Autodesk Fusion 360 part; units mm, degrees
(part 2 of 2)
  arc A18 (-11.9213, -3.7594) -> (-11.7413, -4.2886) centre (0, 0) ccw
  spline S37 degree 5 poles (-11.7413, -4.2886) (-11.7404, -4.3045) (-11.7391, -4.3362) (-11.7389, -4.383) (-11.7421, -4.4438) (-11.7524, -4.517) (-11.7695, -4.5872) (-11.7939, -4.6541) (-11.8261, -4.7177) (-11.8656, -4.778) (-11.9119, -4.8353) (-11.954, -4.8789) (-11.9882, -4.9104) (-12.0121, -4.931) (-12.0244, -4.9411) knots -1 -1 -1 -1 -1 -1 -0.9 -0.8 -0.7 -0.6 -0.5 -0.4 -0.3 -0.2 -0.1 0 0 0 0 0 0
  line L95 (-12.0244, -4.9411) -> (-12.9493, -5.3212)
  line L96 (-12.9493, -5.3212) -> (-14.2037, -6.215)
  line L97 (-14.2037, -6.215) -> (-13.8236, -7.14)
  line L98 (-13.8236, -7.14) -> (-12.2495, -6.8715)
  line L99 (-12.2495, -6.8715) -> (-11.2708, -6.4694)
  spline S38 degree 5 poles (-11.2708, -6.4694) (-11.2543, -6.467) (-11.2214, -6.4628) (-11.1727, -6.4584) (-11.1087, -6.4566) (-11.0305, -6.4612) (-10.9543, -6.4735) (-10.8803, -6.494) (-10.8086, -6.523) (-10.739, -6.5603) (-10.6714, -6.6051) (-10.6188, -6.6465) (-10.5801, -6.6805) (-10.5547, -6.7045) (-10.542, -6.7168) knots 0 0 0 0 0 0 0.1 0.2 0.3 0.4 0.5 0.6 0.7 0.8 0.9 1 1 1 1 1 1
  arc A19 (-10.542, -6.7168) -> (-10.2313, -7.1813) centre (0, 0) ccw
  spline S39 degree 5 poles (-10.2313, -7.1813) (-10.2262, -7.1965) (-10.2168, -7.2268) (-10.2045, -7.2719) (-10.1918, -7.3314) (-10.1828, -7.4048) (-10.1812, -7.477) (-10.1875, -7.548) (-10.2021, -7.6177) (-10.2246, -7.6862) (-10.2546, -7.7535) (-10.2839, -7.8066) (-10.3088, -7.8459) (-10.3266, -7.8719) (-10.3358, -7.8849) knots -1 -1 -1 -1 -1 -1 -0.9 -0.8 -0.7 -0.6 -0.5 -0.4 -0.3 -0.2 -0.1 0 0 0 0 0 0
  line L100 (-10.3358, -7.8849) -> (-11.1309, -8.4914)
  line L101 (-11.1309, -8.4914) -> (-12.1112, -9.6795)
  line L102 (-12.1112, -9.6795) -> (-11.5047, -10.4745)
  line L103 (-11.5047, -10.4745) -> (-10.0536, -9.8078)
  line L104 (-10.0536, -9.8078) -> (-9.2124, -9.166)
  spline S40 degree 5 poles (-9.2124, -9.166) (-9.197, -9.1594) (-9.1664, -9.1469) (-9.1204, -9.1301) (-9.0591, -9.1117) (-8.9823, -9.096) (-8.9056, -9.0881) (-8.8288, -9.0888) (-8.752, -9.0982) (-8.6752, -9.1162) (-8.5983, -9.142) (-8.5367, -9.1684) (-8.4906, -9.1913) (-8.4598, -9.2078) (-8.4444, -9.2164) knots 0 0 0 0 0 0 0.1 0.2 0.3 0.4 0.5 0.6 0.7 0.8 0.9 1 1 1 1 1 1
  arc A20 (-8.4444, -9.2164) -> (-8.024, -9.5847) centre (0, 0) ccw
  spline S41 degree 5 poles (-8.024, -9.5847) (-8.0152, -9.598) (-7.9982, -9.6248) (-7.9747, -9.6652) (-7.9471, -9.7194) (-7.9194, -9.788) (-7.8991, -9.8573) (-7.8868, -9.9276) (-7.8828, -9.9987) (-7.8869, -10.0706) (-7.8984, -10.1434) (-7.913, -10.2022) (-7.9268, -10.2466) (-7.9373, -10.2764) (-7.9429, -10.2913) knots -1 -1 -1 -1 -1 -1 -0.9 -0.8 -0.7 -0.6 -0.5 -0.4 -0.3 -0.2 -0.1 0 0 0 0 0 0
  line L105 (-7.9429, -10.2913) -> (-8.5539, -11.0829)
  line L106 (-8.5539, -11.0829) -> (-9.1933, -12.4842)
  line L107 (-9.1933, -12.4842) -> (-8.4016, -13.0952)
  line L108 (-8.4016, -13.0952) -> (-7.1726, -12.0756)
  line L109 (-7.1726, -12.0756) -> (-6.5261, -11.238)
  spline S42 degree 5 poles (-6.5261, -11.238) (-6.513, -11.2277) (-6.4867, -11.2076) (-6.4466, -11.1795) (-6.3921, -11.1459) (-6.3221, -11.1109) (-6.25, -11.0834) (-6.1756, -11.0641) (-6.099, -11.0534) (-6.0201, -11.0509) (-5.9392, -11.0559) (-5.8729, -11.0655) (-5.8224, -11.0756) (-5.7884, -11.0836) (-5.7713, -11.0879) knots 0 0 0 0 0 0 0.1 0.2 0.3 0.4 0.5 0.6 0.7 0.8 0.9 1 1 1 1 1 1
  arc A21 (-5.7713, -11.0879) -> (-5.2699, -11.3348) centre (0, 0) ccw
  spline S43 degree 5 poles (-5.2699, -11.3348) (-5.2579, -11.3455) (-5.2346, -11.3669) (-5.2014, -11.3998) (-5.1607, -11.4451) (-5.1162, -11.5042) (-5.0786, -11.5659) (-5.0486, -11.6305) (-5.0264, -11.6982) (-5.0117, -11.7688) (-5.0039, -11.842) (-5.0029, -11.9026) (-5.0047, -11.9491) (-5.0071, -11.9806) (-5.0086, -11.9964) knots -1 -1 -1 -1 -1 -1 -0.9 -0.8 -0.7 -0.6 -0.5 -0.4 -0.3 -0.2 -0.1 0 0 0 0 0 0
  line L110 (-5.0086, -11.9964) -> (-5.3939, -12.9192)
  line L111 (-5.3939, -12.9192) -> (-5.6489, -14.4382)
  line L112 (-5.6489, -14.4382) -> (-4.7261, -14.8235)
  line L113 (-4.7261, -14.8235) -> (-3.8028, -13.5206)
  line L114 (-3.8028, -13.5206) -> (-3.3951, -12.5442)
  spline S44 degree 5 poles (-3.3951, -12.5442) (-3.3852, -12.5308) (-3.3649, -12.5046) (-3.3335, -12.4671) (-3.2895, -12.4205) (-3.2309, -12.3685) (-3.1684, -12.3233) (-3.1016, -12.2855) (-3.0303, -12.2553) (-2.9548, -12.2325) (-2.8753, -12.2164) (-2.8088, -12.2085) (-2.7574, -12.2051) (-2.7225, -12.2041) (-2.7049, -12.2038) knots 0 0 0 0 0 0 0.1 0.2 0.3 0.4 0.5 0.6 0.7 0.8 0.9 1 1 1 1 1 1
  arc A22 (-2.7049, -12.2038) -> (-2.1566, -12.3126) centre (0, 0) ccw
  spline S45 degree 5 poles (-2.1566, -12.3126) (-2.1423, -12.3197) (-2.1143, -12.3344) (-2.0737, -12.3576) (-2.0226, -12.3908) (-1.9644, -12.4363) (-1.9121, -12.4862) (-1.8664, -12.5409) (-1.8274, -12.6005) (-1.7949, -12.6649) (-1.7685, -12.7337) (-1.7518, -12.7919) (-1.7415, -12.8373) (-1.7357, -12.8683) (-1.7331, -12.884) knots -1 -1 -1 -1 -1 -1 -0.9 -0.8 -0.7 -0.6 -0.5 -0.4 -0.3 -0.2 -0.1 0 0 0 0 0 0
  line L115 (-1.7331, -12.884) -> (-1.8664, -13.875)
  line L116 (-1.8664, -13.875) -> (-1.7195, -15.4083)
  line L117 (-1.7195, -15.4083) -> (-0.7284, -15.5416)
  line L118 (-0.7284, -15.5416) -> (-0.1738, -14.0441)
  line L119 (-0.1738, -14.0441) -> (0, -12.7519)
  line L120 (0, -12.7519) -> (0, -12.9212)
  spline S46 degree 5 poles (0, -12.9212) (0.0001, -12.921) (0.0073, -12.9063) (0.0221, -12.8775) (0.0458, -12.8358) (0.0804, -12.7833) (0.1291, -12.7235) (0.1838, -12.6697) (0.2448, -12.622) (0.3119, -12.5804) (0.3845, -12.5443) (0.4467, -12.5194) (0.4955, -12.5029) (0.5289, -12.4929) (0.5459, -12.4881) knots 0.098741 0.098741 0.098741 0.098741 0.098741 0.098741 0.1 0.2 0.3 0.4 0.5 0.6 0.7 0.8 0.9 1 1 1 1 1 1
  arc A23 (0.5459, -12.4881) -> (1.1036, -12.4512) centre (0, 0) ccw
  spline S47 degree 5 poles (1.1036, -12.4512) (1.1192, -12.4544) (1.1502, -12.4614) (1.1954, -12.4733) (1.2533, -12.4921) (1.3213, -12.521) (1.3847, -12.5557) (1.443, -12.5966) (1.4961, -12.6441) (1.5441, -12.6979) (1.5875, -12.7575) (1.6187, -12.8094) (1.6403, -12.8506) (1.654, -12.879) (1.6606, -12.8935) knots -1 -1 -1 -1 -1 -1 -0.9 -0.8 -0.7 -0.6 -0.5 -0.4 -0.3 -0.2 -0.1 0 0 0 0 0 0
  line L121 (1.6606, -12.8935) -> (1.7883, -13.8853)
  line L122 (1.7883, -13.8853) -> (2.3271, -15.3283)
  circle A24 centre (0, 0) radius 1.5
  dimension "d23" = 3
  constraint coincident A0.centre A1.centre
  measures "d23" diameter of A24
extrude "Extrude2" cut sketch "Sketch2" against normal blind 10 contours A24
sketch "Sketch3" plane through (0, 4, 0) normal (0, 1, 0) x (-1, 0, 0)
  circle A0 centre (0, 0) radius 1.5
  line L0 (2.3271, -15.3283) -> (3.3189, -15.2006)
  line L1 (3.3189, -15.2006) -> (3.467, -13.6106)
  line L2 (3.467, -13.6106) -> (3.3318, -12.5612)
  spline S0 degree 5 poles (3.3318, -12.5612) (3.3338, -12.5446) (3.3382, -12.5118) (3.3467, -12.4635) (3.3614, -12.4012) (3.3862, -12.3269) (3.4177, -12.2565) (3.4567, -12.1904) (3.5033, -12.1286) (3.5573, -12.071) (3.6181, -12.0173) (3.6717, -11.9772) (3.7146, -11.9487) (3.7443, -11.9303) (3.7594, -11.9213) knots 0 0 0 0 0 0 0.1 0.2 0.3 0.4 0.5 0.6 0.7 0.8 0.9 1 1 1 1 1 1
  arc A1 (3.7594, -11.9213) -> (4.751, -11.5619) centre (0, 0) ccw
  line L3 (4.751, -11.5619) -> (4.3177, -11.74)
  spline S1 degree 5 poles (4.3177, -11.74) (4.3277, -11.7396) (4.3533, -11.7391) (4.3941, -11.7395) (4.4491, -11.7428) (4.517, -11.7524) (4.5872, -11.7695) (4.6541, -11.7939) (4.7177, -11.8261) (4.778, -11.8656) (4.8353, -11.9119) (4.8789, -11.954) (4.9104, -11.9882) (4.931, -12.0121) (4.9411, -12.0244) knots -0.963292 -0.963292 -0.963292 -0.963292 -0.963292 -0.963292 -0.9 -0.8 -0.7 -0.6 -0.5 -0.4 -0.3 -0.2 -0.1 0 0 0 0 0 0
  line L4 (4.9411, -12.0244) -> (5.3212, -12.9493)
  line L5 (5.3212, -12.9493) -> (6.215, -14.2037)
  line L6 (6.215, -14.2037) -> (7.14, -13.8236)
  line L7 (7.14, -13.8236) -> (6.8715, -12.2495)
  line L8 (6.8715, -12.2495) -> (6.4694, -11.2708)
  spline S2 degree 5 poles (6.4694, -11.2708) (6.467, -11.2543) (6.4628, -11.2214) (6.4584, -11.1727) (6.4566, -11.1087) (6.4612, -11.0305) (6.4735, -10.9543) (6.494, -10.8803) (6.523, -10.8086) (6.5603, -10.739) (6.6013, -10.6771) (6.6378, -10.63) (6.6663, -10.5966) (6.6845, -10.5763) (6.6913, -10.569) knots 0 0 0 0 0 0 0.1 0.2 0.3 0.4 0.5 0.6 0.7 0.8 0.9 0.957627 0.957627 0.957627 0.957627 0.957627 0.957627
  line L9 (6.6913, -10.569) -> (6.2793, -10.8083)
  arc A2 (6.2793, -10.8083) -> (7.1813, -10.2313) centre (0, 0) ccw
  spline S3 degree 5 poles (7.1813, -10.2313) (7.1965, -10.2262) (7.2268, -10.2168) (7.2719, -10.2045) (7.3314, -10.1918) (7.4048, -10.1828) (7.477, -10.1812) (7.548, -10.1875) (7.6177, -10.2021) (7.6862, -10.2246) (7.7535, -10.2546) (7.8066, -10.2839) (7.8459, -10.3088) (7.8719, -10.3266) (7.8849, -10.3358) knots -1 -1 -1 -1 -1 -1 -0.9 -0.8 -0.7 -0.6 -0.5 -0.4 -0.3 -0.2 -0.1 0 0 0 0 0 0
  line L10 (7.8849, -10.3358) -> (8.4914, -11.1309)
  line L11 (8.4914, -11.1309) -> (9.6795, -12.1112)
  line L12 (9.6795, -12.1112) -> (10.4745, -11.5047)
  line L13 (10.4745, -11.5047) -> (9.8078, -10.0536)
  line L14 (9.8078, -10.0536) -> (9.166, -9.2124)
  spline S4 degree 5 poles (9.166, -9.2124) (9.1594, -9.197) (9.1469, -9.1664) (9.1301, -9.1204) (9.1117, -9.0591) (9.096, -8.9823) (9.0881, -8.9056) (9.0888, -8.8288) (9.0982, -8.752) (9.1162, -8.6752) (9.142, -8.5983) (9.1684, -8.5367) (9.1913, -8.4906) (9.2078, -8.4598) (9.2164, -8.4444) knots 0 0 0 0 0 0 0.1 0.2 0.3 0.4 0.5 0.6 0.7 0.8 0.9 1 1 1 1 1 1
  arc A3 (9.2164, -8.4444) -> (9.5847, -8.024) centre (0, 0) ccw
  spline S5 degree 5 poles (9.5847, -8.024) (9.598, -8.0152) (9.6248, -7.9982) (9.6652, -7.9747) (9.7194, -7.9471) (9.788, -7.9194) (9.8573, -7.8991) (9.9276, -7.8868) (9.9987, -7.8828) (10.0706, -7.8869) (10.1434, -7.8984) (10.2022, -7.913) (10.2466, -7.9268) (10.2764, -7.9373) (10.2913, -7.9429) knots -1 -1 -1 -1 -1 -1 -0.9 -0.8 -0.7 -0.6 -0.5 -0.4 -0.3 -0.2 -0.1 0 0 0 0 0 0
  line L15 (10.2913, -7.9429) -> (11.0829, -8.5539)
  line L16 (11.0829, -8.5539) -> (12.4842, -9.1933)
  line L17 (12.4842, -9.1933) -> (13.0952, -8.4016)
  line L18 (13.0952, -8.4016) -> (12.0756, -7.1726)
  line L19 (12.0756, -7.1726) -> (11.238, -6.5261)
  spline S6 degree 5 poles (11.238, -6.5261) (11.2277, -6.513) (11.2076, -6.4867) (11.1795, -6.4466) (11.1459, -6.3921) (11.1109, -6.3221) (11.0834, -6.25) (11.0641, -6.1756) (11.0534, -6.099) (11.0509, -6.0201) (11.0559, -5.9392) (11.0655, -5.8729) (11.0756, -5.8224) (11.0836, -5.7884) (11.0879, -5.7713) knots 0 0 0 0 0 0 0.1 0.2 0.3 0.4 0.5 0.6 0.7 0.8 0.9 1 1 1 1 1 1
  arc A4 (11.0879, -5.7713) -> (11.3348, -5.2699) centre (0, 0) ccw
  spline S7 degree 5 poles (11.3348, -5.2699) (11.3455, -5.2579) (11.3669, -5.2346) (11.3998, -5.2014) (11.4451, -5.1607) (11.5042, -5.1162) (11.5659, -5.0786) (11.6305, -5.0486) (11.6982, -5.0264) (11.7688, -5.0117) (11.842, -5.0039) (11.9026, -5.0029) (11.9491, -5.0047) (11.9806, -5.0071) (11.9964, -5.0086) knots -1 -1 -1 -1 -1 -1 -0.9 -0.8 -0.7 -0.6 -0.5 -0.4 -0.3 -0.2 -0.1 0 0 0 0 0 0
  line L20 (11.9964, -5.0086) -> (12.9192, -5.3939)
  line L21 (12.9192, -5.3939) -> (14.4382, -5.6489)
  line L22 (14.4382, -5.6489) -> (14.8235, -4.7261)
  line L23 (14.8235, -4.7261) -> (13.5206, -3.8028)
  line L24 (13.5206, -3.8028) -> (12.5442, -3.3951)
  spline S8 degree 5 poles (12.5442, -3.3951) (12.5308, -3.3852) (12.5046, -3.3649) (12.4671, -3.3335) (12.4205, -3.2895) (12.3685, -3.2309) (12.3233, -3.1684) (12.2855, -3.1016) (12.2553, -3.0303) (12.2325, -2.9548) (12.2164, -2.8753) (12.2085, -2.8088) (12.2051, -2.7574) (12.2041, -2.7225) (12.2038, -2.7049) knots 0 0 0 0 0 0 0.1 0.2 0.3 0.4 0.5 0.6 0.7 0.8 0.9 1 1 1 1 1 1
  arc A5 (12.2038, -2.7049) -> (12.3126, -2.1566) centre (0, 0) ccw
  spline S9 degree 5 poles (12.3126, -2.1566) (12.3197, -2.1423) (12.3344, -2.1143) (12.3576, -2.0737) (12.3908, -2.0226) (12.4363, -1.9644) (12.4862, -1.9121) (12.5409, -1.8664) (12.6005, -1.8274) (12.6649, -1.7949) (12.7337, -1.7685) (12.7919, -1.7518) (12.8373, -1.7415) (12.8683, -1.7357) (12.884, -1.7331) knots -1 -1 -1 -1 -1 -1 -0.9 -0.8 -0.7 -0.6 -0.5 -0.4 -0.3 -0.2 -0.1 0 0 0 0 0 0
  line L25 (12.884, -1.7331) -> (13.875, -1.8664)
  line L26 (13.875, -1.8664) -> (15.4083, -1.7195)
  line L27 (15.4083, -1.7195) -> (15.5416, -0.7284)
  line L28 (15.5416, -0.7284) -> (14.0441, -0.1738)
  line L29 (14.0441, -0.1738) -> (12.9955, -0.0328)
  spline S10 degree 5 poles (12.9955, -0.0328) (12.98, -0.0266) (12.9494, -0.0138) (12.905, 0.0068) (12.8487, 0.0372) (12.7833, 0.0804) (12.7235, 0.1291) (12.6697, 0.1838) (12.622, 0.2448) (12.5804, 0.3119) (12.5443, 0.3845) (12.5194, 0.4467) (12.5029, 0.4955) (12.4929, 0.5289) (12.4881, 0.5459) knots 0 0 0 0 0 0 0.1 0.2 0.3 0.4 0.5 0.6 0.7 0.8 0.9 1 1 1 1 1 1
  arc A6 (12.4881, 0.5459) -> (12.4512, 1.1036) centre (0, 0) ccw
  spline S11 degree 5 poles (12.4512, 1.1036) (12.4544, 1.1192) (12.4614, 1.1502) (12.4733, 1.1954) (12.4921, 1.2533) (12.521, 1.3213) (12.5557, 1.3847) (12.5966, 1.443) (12.6441, 1.4961) (12.6979, 1.5441) (12.7575, 1.5875) (12.8094, 1.6187) (12.8506, 1.6403) (12.879, 1.654) (12.8935, 1.6606) knots -1 -1 -1 -1 -1 -1 -0.9 -0.8 -0.7 -0.6 -0.5 -0.4 -0.3 -0.2 -0.1 0 0 0 0 0 0
  line L30 (12.8935, 1.6606) -> (13.8853, 1.7883)
  line L31 (13.8853, 1.7883) -> (15.3283, 2.3271)
  line L32 (15.3283, 2.3271) -> (15.2006, 3.3189)
  line L33 (15.2006, 3.3189) -> (13.6106, 3.467)
  line L34 (13.6106, 3.467) -> (12.5612, 3.3318)
  spline S12 degree 5 poles (12.5612, 3.3318) (12.5446, 3.3338) (12.5118, 3.3382) (12.4635, 3.3467) (12.4012, 3.3614) (12.3269, 3.3862) (12.2565, 3.4177) (12.1904, 3.4567) (12.1286, 3.5033) (12.071, 3.5573) (12.0173, 3.6181) (11.9772, 3.6717) (11.9487, 3.7146) (11.9303, 3.7443) (11.9213, 3.7594) knots 0 0 0 0 0 0 0.1 0.2 0.3 0.4 0.5 0.6 0.7 0.8 0.9 1 1 1 1 1 1
  arc A7 (11.9213, 3.7594) -> (11.7413, 4.2886) centre (0, 0) ccw
  spline S13 degree 5 poles (11.7413, 4.2886) (11.7404, 4.3045) (11.7391, 4.3362) (11.7389, 4.383) (11.7421, 4.4438) (11.7524, 4.517) (11.7695, 4.5872) (11.7939, 4.6541) (11.8261, 4.7177) (11.8656, 4.778) (11.9119, 4.8353) (11.954, 4.8789) (11.9882, 4.9104) (12.0121, 4.931) (12.0244, 4.9411) knots -1 -1 -1 -1 -1 -1 -0.9 -0.8 -0.7 -0.6 -0.5 -0.4 -0.3 -0.2 -0.1 0 0 0 0 0 0
  line L35 (12.0244, 4.9411) -> (12.9493, 5.3212)
  line L36 (12.9493, 5.3212) -> (14.2037, 6.215)
  line L37 (14.2037, 6.215) -> (13.8236, 7.14)
  line L38 (13.8236, 7.14) -> (12.2495, 6.8715)
  line L39 (12.2495, 6.8715) -> (11.2708, 6.4694)
  spline S14 degree 5 poles (11.2708, 6.4694) (11.2543, 6.467) (11.2214, 6.4628) (11.1727, 6.4584) (11.1087, 6.4566) (11.0305, 6.4612) (10.9543, 6.4735) (10.8803, 6.494) (10.8086, 6.523) (10.739, 6.5603) (10.6714, 6.6051) (10.6188, 6.6465) (10.5801, 6.6805) (10.5547, 6.7045) (10.542, 6.7168) knots 0 0 0 0 0 0 0.1 0.2 0.3 0.4 0.5 0.6 0.7 0.8 0.9 1 1 1 1 1 1
  arc A8 (10.542, 6.7168) -> (10.2313, 7.1813) centre (0, 0) ccw
  spline S15 degree 5 poles (10.2313, 7.1813) (10.2262, 7.1965) (10.2168, 7.2268) (10.2045, 7.2719) (10.1918, 7.3314) (10.1828, 7.4048) (10.1812, 7.477) (10.1875, 7.548) (10.2021, 7.6177) (10.2246, 7.6862) (10.2546, 7.7535) (10.2839, 7.8066) (10.3088, 7.8459) (10.3266, 7.8719) (10.3358, 7.8849) knots -1 -1 -1 -1 -1 -1 -0.9 -0.8 -0.7 -0.6 -0.5 -0.4 -0.3 -0.2 -0.1 0 0 0 0 0 0
  line L40 (10.3358, 7.8849) -> (11.1309, 8.4914)
  line L41 (11.1309, 8.4914) -> (12.1112, 9.6795)
  line L42 (12.1112, 9.6795) -> (11.5047, 10.4745)
  line L43 (11.5047, 10.4745) -> (10.0536, 9.8078)
  line L44 (10.0536, 9.8078) -> (9.2124, 9.166)
  spline S16 degree 5 poles (9.2124, 9.166) (9.197, 9.1594) (9.1664, 9.1469) (9.1204, 9.1301) (9.0591, 9.1117) (8.9823, 9.096) (8.9056, 9.0881) (8.8288, 9.0888) (8.752, 9.0982) (8.6752, 9.1162) (8.5983, 9.142) (8.5367, 9.1684) (8.4906, 9.1913) (8.4598, 9.2078) (8.4444, 9.2164) knots 0 0 0 0 0 0 0.1 0.2 0.3 0.4 0.5 0.6 0.7 0.8 0.9 1 1 1 1 1 1
  arc A9 (8.4444, 9.2164) -> (8.024, 9.5847) centre (0, 0) ccw
  spline S17 degree 5 poles (8.024, 9.5847) (8.0152, 9.598) (7.9982, 9.6248) (7.9747, 9.6652) (7.9471, 9.7194) (7.9194, 9.788) (7.8991, 9.8573) (7.8868, 9.9276) (7.8828, 9.9987) (7.8869, 10.0706) (7.8984, 10.1434) (7.913, 10.2022) (7.9268, 10.2466) (7.9373, 10.2764) (7.9429, 10.2913) knots -1 -1 -1 -1 -1 -1 -0.9 -0.8 -0.7 -0.6 -0.5 -0.4 -0.3 -0.2 -0.1 0 0 0 0 0 0
  line L45 (7.9429, 10.2913) -> (8.5539, 11.0829)
  line L46 (8.5539, 11.0829) -> (9.1933, 12.4842)
  line L47 (9.1933, 12.4842) -> (8.4016, 13.0952)
  line L48 (8.4016, 13.0952) -> (7.1726, 12.0756)
  line L49 (7.1726, 12.0756) -> (6.5261, 11.238)
  spline S18 degree 5 poles (6.5261, 11.238) (6.513, 11.2277) (6.4867, 11.2076) (6.4466, 11.1795) (6.3921, 11.1459) (6.3221, 11.1109) (6.25, 11.0834) (6.1756, 11.0641) (6.099, 11.0534) (6.0201, 11.0509) (5.9392, 11.0559) (5.8729, 11.0655) (5.8224, 11.0756) (5.7884, 11.0836) (5.7713, 11.0879) knots 0 0 0 0 0 0 0.1 0.2 0.3 0.4 0.5 0.6 0.7 0.8 0.9 1 1 1 1 1 1
  arc A10 (5.7713, 11.0879) -> (5.2699, 11.3348) centre (0, 0) ccw
  spline S19 degree 5 poles (5.2699, 11.3348) (5.2579, 11.3455) (5.2346, 11.3669) (5.2014, 11.3998) (5.1607, 11.4451) (5.1162, 11.5042) (5.0786, 11.5659) (5.0486, 11.6305) (5.0264, 11.6982) (5.0117, 11.7688) (5.0039, 11.842) (5.0029, 11.9026) (5.0047, 11.9491) (5.0071, 11.9806) (5.0086, 11.9964) knots -1 -1 -1 -1 -1 -1 -0.9 -0.8 -0.7 -0.6 -0.5 -0.4 -0.3 -0.2 -0.1 0 0 0 0 0 0
  line L50 (5.0086, 11.9964) -> (5.3939, 12.9192)
  line L51 (5.3939, 12.9192) -> (5.6489, 14.4382)
  line L52 (5.6489, 14.4382) -> (4.7261, 14.8235)
  line L53 (4.7261, 14.8235) -> (3.8028, 13.5206)
  line L54 (3.8028, 13.5206) -> (3.3951, 12.5442)
  spline S20 degree 5 poles (3.3951, 12.5442) (3.3852, 12.5308) (3.3649, 12.5046) (3.3335, 12.4671) (3.2895, 12.4205) (3.2309, 12.3685) (3.1684, 12.3233) (3.1016, 12.2855) (3.0303, 12.2553) (2.9548, 12.2325) (2.8753, 12.2164) (2.8088, 12.2085) (2.7574, 12.2051) (2.7225, 12.2041) (2.7049, 12.2038) knots 0 0 0 0 0 0 0.1 0.2 0.3 0.4 0.5 0.6 0.7 0.8 0.9 1 1 1 1 1 1
  arc A11 (2.7049, 12.2038) -> (2.1566, 12.3126) centre (0, 0) ccw
  spline S21 degree 5 poles (2.1566, 12.3126) (2.1423, 12.3197) (2.1143, 12.3344) (2.0737, 12.3576) (2.0226, 12.3908) (1.9644, 12.4363) (1.9121, 12.4862) (1.8664, 12.5409) (1.8274, 12.6005) (1.7949, 12.6649) (1.7685, 12.7337) (1.7518, 12.7919) (1.7415, 12.8373) (1.7357, 12.8683) (1.7331, 12.884) knots -1 -1 -1 -1 -1 -1 -0.9 -0.8 -0.7 -0.6 -0.5 -0.4 -0.3 -0.2 -0.1 0 0 0 0 0 0
  line L55 (1.7331, 12.884) -> (1.8664, 13.875)
  line L56 (1.8664, 13.875) -> (1.7195, 15.4083)
  line L57 (1.7195, 15.4083) -> (0.7284, 15.5416)
  line L58 (0.7284, 15.5416) -> (0.1738, 14.0441)
  line L59 (0.1738, 14.0441) -> (0.0328, 12.9955)
  spline S22 degree 5 poles (0.0328, 12.9955) (0.0266, 12.98) (0.0138, 12.9494) (-0.0068, 12.905) (-0.0372, 12.8487) (-0.0804, 12.7833) (-0.1291, 12.7235) (-0.1838, 12.6697) (-0.2448, 12.622) (-0.3119, 12.5804) (-0.3845, 12.5443) (-0.4467, 12.5194) (-0.4955, 12.5029) (-0.5289, 12.4929) (-0.5459, 12.4881) knots 0 0 0 0 0 0 0.1 0.2 0.3 0.4 0.5 0.6 0.7 0.8 0.9 1 1 1 1 1 1
  arc A12 (-0.5459, 12.4881) -> (-1.1036, 12.4512) centre (0, 0) ccw
  spline S23 degree 5 poles (-1.1036, 12.4512) (-1.1192, 12.4544) (-1.1502, 12.4614) (-1.1954, 12.4733) (-1.2533, 12.4921) (-1.3213, 12.521) (-1.3847, 12.5557) (-1.443, 12.5966) (-1.4961, 12.6441) (-1.5441, 12.6979) (-1.5875, 12.7575) (-1.6187, 12.8094) (-1.6403, 12.8506) (-1.654, 12.879) (-1.6606, 12.8935) knots -1 -1 -1 -1 -1 -1 -0.9 -0.8 -0.7 -0.6 -0.5 -0.4 -0.3 -0.2 -0.1 0 0 0 0 0 0
  line L60 (-1.6606, 12.8935) -> (-1.7883, 13.8853)
  line L61 (-1.7883, 13.8853) -> (-2.3271, 15.3283)
  line L62 (-2.3271, 15.3283) -> (-3.3189, 15.2006)
  line L63 (-3.3189, 15.2006) -> (-3.467, 13.6106)
  line L64 (-3.467, 13.6106) -> (-3.3318, 12.5612)
  spline S24 degree 5 poles (-3.3318, 12.5612) (-3.3338, 12.5446) (-3.3382, 12.5118) (-3.3467, 12.4635) (-3.3614, 12.4012) (-3.3862, 12.3269) (-3.4177, 12.2565) (-3.4567, 12.1904) (-3.5033, 12.1286) (-3.5573, 12.071) (-3.6181, 12.0173) (-3.6717, 11.9772) (-3.7146, 11.9487) (-3.7443, 11.9303) (-3.7594, 11.9213) knots 0 0 0 0 0 0 0.1 0.2 0.3 0.4 0.5 0.6 0.7 0.8 0.9 1 1 1 1 1 1
  arc A13 (-3.7594, 11.9213) -> (-4.2886, 11.7413) centre (0, 0) ccw
  spline S25 degree 5 poles (-4.2886, 11.7413) (-4.3045, 11.7404) (-4.3362, 11.7391) (-4.383, 11.7389) (-4.4438, 11.7421) (-4.517, 11.7524) (-4.5872, 11.7695) (-4.6541, 11.7939) (-4.7177, 11.8261) (-4.778, 11.8656) (-4.8353, 11.9119) (-4.8789, 11.954) (-4.9104, 11.9882) (-4.931, 12.0121) (-4.9411, 12.0244) knots -1 -1 -1 -1 -1 -1 -0.9 -0.8 -0.7 -0.6 -0.5 -0.4 -0.3 -0.2 -0.1 0 0 0 0 0 0
  line L65 (-4.9411, 12.0244) -> (-5.3212, 12.9493)
  line L66 (-5.3212, 12.9493) -> (-6.215, 14.2037)
  line L67 (-6.215, 14.2037) -> (-7.14, 13.8236)
  line L68 (-7.14, 13.8236) -> (-6.8715, 12.2495)
  line L69 (-6.8715, 12.2495) -> (-6.4694, 11.2708)
  spline S26 degree 5 poles (-6.4694, 11.2708) (-6.467, 11.2543) (-6.4628, 11.2214) (-6.4584, 11.1727) (-6.4566, 11.1087) (-6.4612, 11.0305) (-6.4735, 10.9543) (-6.494, 10.8803) (-6.523, 10.8086) (-6.5603, 10.739) (-6.6051, 10.6714) (-6.6465, 10.6188) (-6.6805, 10.5801) (-6.7045, 10.5547) (-6.7168, 10.542) knots 0 0 0 0 0 0 0.1 0.2 0.3 0.4 0.5 0.6 0.7 0.8 0.9 1 1 1 1 1 1
  arc A14 (-6.7168, 10.542) -> (-7.1813, 10.2313) centre (0, 0) ccw
  spline S27 degree 5 poles (-7.1813, 10.2313) (-7.1965, 10.2262) (-7.2268, 10.2168) (-7.2719, 10.2045) (-7.3314, 10.1918) (-7.4048, 10.1828) (-7.477, 10.1812) (-7.548, 10.1875) (-7.6177, 10.2021) (-7.6862, 10.2246) (-7.7535, 10.2546) (-7.8066, 10.2839) (-7.8459, 10.3088) (-7.8719, 10.3266) (-7.8849, 10.3358) knots -1 -1 -1 -1 -1 -1 -0.9 -0.8 -0.7 -0.6 -0.5 -0.4 -0.3 -0.2 -0.1 0 0 0 0 0 0
  line L70 (-7.8849, 10.3358) -> (-8.4914, 11.1309)
  line L71 (-8.4914, 11.1309) -> (-9.6795, 12.1112)
  line L72 (-9.6795, 12.1112) -> (-10.4745, 11.5047)
  line L73 (-10.4745, 11.5047) -> (-9.8078, 10.0536)
  line L74 (-9.8078, 10.0536) -> (-9.166, 9.2124)
  spline S28 degree 5 poles (-9.166, 9.2124) (-9.1594, 9.197) (-9.1469, 9.1664) (-9.1301, 9.1204) (-9.1117, 9.0591) (-9.096, 8.9823) (-9.0881, 8.9056) (-9.0888, 8.8288) (-9.0982, 8.752) (-9.1162, 8.6752) (-9.142, 8.5983) (-9.1684, 8.5367) (-9.1913, 8.4906) (-9.2078, 8.4598) (-9.2164, 8.4444) knots 0 0 0 0 0 0 0.1 0.2 0.3 0.4 0.5 0.6 0.7 0.8 0.9 1 1 1 1 1 1
  arc A15 (-9.2164, 8.4444) -> (-9.5847, 8.024) centre (0, 0) ccw
  spline S29 degree 5 poles (-9.5847, 8.024) (-9.598, 8.0152) (-9.6248, 7.9982) (-9.6652, 7.9747) (-9.7194, 7.9471) (-9.788, 7.9194) (-9.8573, 7.8991) (-9.9276, 7.8868) (-9.9987, 7.8828) (-10.0706, 7.8869) (-10.1434, 7.8984) (-10.2022, 7.913) (-10.2466, 7.9268) (-10.2764, 7.9373) (-10.2913, 7.9429) knots -1 -1 -1 -1 -1 -1 -0.9 -0.8 -0.7 -0.6 -0.5 -0.4 -0.3 -0.2 -0.1 0 0 0 0 0 0
  line L75 (-10.2913, 7.9429) -> (-11.0829, 8.5539)
  line L76 (-11.0829, 8.5539) -> (-12.4842, 9.1933)
  line L77 (-12.4842, 9.1933) -> (-13.0952, 8.4016)
  line L78 (-13.0952, 8.4016) -> (-12.0756, 7.1726)
  line L79 (-12.0756, 7.1726) -> (-11.238, 6.5261)
  spline S30 degree 5 poles (-11.238, 6.5261) (-11.2277, 6.513) (-11.2076, 6.4867) (-11.1795, 6.4466) (-11.1459, 6.3921) (-11.1109, 6.3221) (-11.0834, 6.25) (-11.0641, 6.1756) (-11.0534, 6.099) (-11.0509, 6.0201) (-11.0559, 5.9392) (-11.0655, 5.8729) (-11.0756, 5.8224) (-11.0836, 5.7884) (-11.0879, 5.7713) knots 0 0 0 0 0 0 0.1 0.2 0.3 0.4 0.5 0.6 0.7 0.8 0.9 1 1 1 1 1 1
  arc A16 (-11.0879, 5.7713) -> (-11.3348, 5.2699) centre (0, 0) ccw
  spline S31 degree 5 poles (-11.3348, 5.2699) (-11.3455, 5.2579) (-11.3669, 5.2346) (-11.3998, 5.2014) (-11.4451, 5.1607) (-11.5042, 5.1162) (-11.5659, 5.0786) (-11.6305, 5.0486) (-11.6982, 5.0264) (-11.7688, 5.0117) (-11.842, 5.0039) (-11.9026, 5.0029) (-11.9491, 5.0047) (-11.9806, 5.0071) (-11.9964, 5.0086) knots -1 -1 -1 -1 -1 -1 -0.9 -0.8 -0.7 -0.6 -0.5 -0.4 -0.3 -0.2 -0.1 0 0 0 0 0 0
  line L80 (-11.9964, 5.0086) -> (-12.9192, 5.3939)
  line L81 (-12.9192, 5.3939) -> (-14.4382, 5.6489)
  line L82 (-14.4382, 5.6489) -> (-14.8235, 4.7261)
  line L83 (-14.8235, 4.7261) -> (-13.5206, 3.8028)
  line L84 (-13.5206, 3.8028) -> (-12.5442, 3.3951)
  spline S32 degree 5 poles (-12.5442, 3.3951) (-12.5308, 3.3852) (-12.5046, 3.3649) (-12.4671, 3.3335) (-12.4205, 3.2895) (-12.3685, 3.2309) (-12.3233, 3.1684) (-12.2855, 3.1016) (-12.2553, 3.0303) (-12.2325, 2.9548) (-12.2164, 2.8753) (-12.2085, 2.8088) (-12.2051, 2.7574) (-12.2041, 2.7225) (-12.2038, 2.7049) knots 0 0 0 0 0 0 0.1 0.2 0.3 0.4 0.5 0.6 0.7 0.8 0.9 1 1 1 1 1 1
  arc A17 (-12.2038, 2.7049) -> (-12.3126, 2.1566) centre (0, 0) ccw
  spline S33 degree 5 poles (-12.3126, 2.1566) (-12.3197, 2.1423) (-12.3344, 2.1143) (-12.3576, 2.0737) (-12.3908, 2.0226) (-12.4363, 1.9644) (-12.4862, 1.9121) (-12.5409, 1.8664) (-12.6005, 1.8274) (-12.6649, 1.7949) (-12.7337, 1.7685) (-12.7919, 1.7518) (-12.8373, 1.7415) (-12.8683, 1.7357) (-12.884, 1.7331) knots -1 -1 -1 -1 -1 -1 -0.9 -0.8 -0.7 -0.6 -0.5 -0.4 -0.3 -0.2 -0.1 0 0 0 0 0 0
  line L85 (-12.884, 1.7331) -> (-13.875, 1.8664)
  line L86 (-13.875, 1.8664) -> (-15.4083, 1.7195)
  line L87 (-15.4083, 1.7195) -> (-15.5416, 0.7284)
  line L88 (-15.5416, 0.7284) -> (-14.0441, 0.1738)
  line L89 (-14.0441, 0.1738) -> (-12.9955, 0.0328)
  spline S34 degree 5 poles (-12.9955, 0.0328) (-12.98, 0.0266) (-12.9494, 0.0138) (-12.905, -0.0068) (-12.8487, -0.0372) (-12.7833, -0.0804) (-12.7235, -0.1291) (-12.6697, -0.1838) (-12.622, -0.2448) (-12.5804, -0.3119) (-12.5443, -0.3845) (-12.5194, -0.4467) (-12.5029, -0.4955) (-12.4929, -0.5289) (-12.4881, -0.5459) knots 0 0 0 0 0 0 0.1 0.2 0.3 0.4 0.5 0.6 0.7 0.8 0.9 1 1 1 1 1 1
  arc A18 (-12.4881, -0.5459) -> (-12.4512, -1.1036) centre (0, 0) ccw
  spline S35 degree 5 poles (-12.4512, -1.1036) (-12.4544, -1.1192) (-12.4614, -1.1502) (-12.4733, -1.1954) (-12.4921, -1.2533) (-12.521, -1.3213) (-12.5557, -1.3847) (-12.5966, -1.443) (-12.6441, -1.4961) (-12.6979, -1.5441) (-12.7575, -1.5875) (-12.8094, -1.6187) (-12.8506, -1.6403) (-12.879, -1.654) (-12.8935, -1.6606) knots -1 -1 -1 -1 -1 -1 -0.9 -0.8 -0.7 -0.6 -0.5 -0.4 -0.3 -0.2 -0.1 0 0 0 0 0 0
  line L90 (-12.8935, -1.6606) -> (-13.8853, -1.7883)
  line L91 (-13.8853, -1.7883) -> (-15.3283, -2.3271)
  line L92 (-15.3283, -2.3271) -> (-15.2006, -3.3189)
  line L93 (-15.2006, -3.3189) -> (-13.6106, -3.467)
  line L94 (-13.6106, -3.467) -> (-12.5612, -3.3318)
  spline S36 degree 5 poles (-12.5612, -3.3318) (-12.5446, -3.3338) (-12.5118, -3.3382) (-12.4635, -3.3467) (-12.4012, -3.3614) (-12.3269, -3.3862) (-12.2565, -3.4177) (-12.1904, -3.4567) (-12.1286, -3.5033) (-12.071, -3.5573) (-12.0173, -3.6181) (-11.9772, -3.6717) (-11.9487, -3.7146) (-11.9303, -3.7443) (-11.9213, -3.7594) knots 0 0 0 0 0 0 0.1 0.2 0.3 0.4 0.5 0.6 0.7 0.8 0.9 1 1 1 1 1 1
  arc A19 (-11.9213, -3.7594) -> (-11.7413, -4.2886) centre (0, 0) ccw
  spline S37 degree 5 poles (-11.7413, -4.2886) (-11.7404, -4.3045) (-11.7391, -4.3362) (-11.7389, -4.383) (-11.7421, -4.4438) (-11.7524, -4.517) (-11.7695, -4.5872) (-11.7939, -4.6541) (-11.8261, -4.7177) (-11.8656, -4.778) (-11.9119, -4.8353) (-11.954, -4.8789) (-11.9882, -4.9104) (-12.0121, -4.931) (-12.0244, -4.9411) knots -1 -1 -1 -1 -1 -1 -0.9 -0.8 -0.7 -0.6 -0.5 -0.4 -0.3 -0.2 -0.1 0 0 0 0 0 0
  line L95 (-12.0244, -4.9411) -> (-12.9493, -5.3212)
  line L96 (-12.9493, -5.3212) -> (-14.2037, -6.215)
  line L97 (-14.2037, -6.215) -> (-13.8236, -7.14)
  line L98 (-13.8236, -7.14) -> (-12.2495, -6.8715)
  line L99 (-12.2495, -6.8715) -> (-11.2708, -6.4694)
  spline S38 degree 5 poles (-11.2708, -6.4694) (-11.2543, -6.467) (-11.2214, -6.4628) (-11.1727, -6.4584) (-11.1087, -6.4566) (-11.0305, -6.4612) (-10.9543, -6.4735) (-10.8803, -6.494) (-10.8086, -6.523) (-10.739, -6.5603) (-10.6714, -6.6051) (-10.6188, -6.6465) (-10.5801, -6.6805) (-10.5547, -6.7045) (-10.542, -6.7168) knots 0 0 0 0 0 0 0.1 0.2 0.3 0.4 0.5 0.6 0.7 0.8 0.9 1 1 1 1 1 1
  arc A20 (-10.542, -6.7168) -> (-10.2313, -7.1813) centre (0, 0) ccw
  spline S39 degree 5 poles (-10.2313, -7.1813) (-10.2262, -7.1965) (-10.2168, -7.2268) (-10.2045, -7.2719) (-10.1918, -7.3314) (-10.1828, -7.4048) (-10.1812, -7.477) (-10.1875, -7.548) (-10.2021, -7.6177) (-10.2246, -7.6862) (-10.2546, -7.7535) (-10.2839, -7.8066) (-10.3088, -7.8459) (-10.3266, -7.8719) (-10.3358, -7.8849) knots -1 -1 -1 -1 -1 -1 -0.9 -0.8 -0.7 -0.6 -0.5 -0.4 -0.3 -0.2 -0.1 0 0 0 0 0 0
  line L100 (-10.3358, -7.8849) -> (-11.1309, -8.4914)
  line L101 (-11.1309, -8.4914) -> (-12.1112, -9.6795)
  line L102 (-12.1112, -9.6795) -> (-11.5047, -10.4745)
  line L103 (-11.5047, -10.4745) -> (-10.0536, -9.8078)
  line L104 (-10.0536, -9.8078) -> (-9.2124, -9.166)
  spline S40 degree 5 poles (-9.2124, -9.166) (-9.197, -9.1594) (-9.1664, -9.1469) (-9.1204, -9.1301) (-9.0591, -9.1117) (-8.9823, -9.096) (-8.9056, -9.0881) (-8.8288, -9.0888) (-8.752, -9.0982) (-8.6752, -9.1162) (-8.5983, -9.142) (-8.5367, -9.1684) (-8.4906, -9.1913) (-8.4598, -9.2078) (-8.4444, -9.2164) knots 0 0 0 0 0 0 0.1 0.2 0.3 0.4 0.5 0.6 0.7 0.8 0.9 1 1 1 1 1 1
  arc A21 (-8.4444, -9.2164) -> (-8.024, -9.5847) centre (0, 0) ccw
  spline S41 degree 5 poles (-8.024, -9.5847) (-8.0152, -9.598) (-7.9982, -9.6248) (-7.9747, -9.6652) (-7.9471, -9.7194) (-7.9194, -9.788) (-7.8991, -9.8573) (-7.8868, -9.9276) (-7.8828, -9.9987) (-7.8869, -10.0706) (-7.8984, -10.1434) (-7.913, -10.2022) (-7.9268, -10.2466) (-7.9373, -10.2764) (-7.9429, -10.2913) knots -1 -1 -1 -1 -1 -1 -0.9 -0.8 -0.7 -0.6 -0.5 -0.4 -0.3 -0.2 -0.1 0 0 0 0 0 0
  line L105 (-7.9429, -10.2913) -> (-8.5539, -11.0829)
  line L106 (-8.5539, -11.0829) -> (-9.1933, -12.4842)
  line L107 (-9.1933, -12.4842) -> (-8.4016, -13.0952)
  line L108 (-8.4016, -13.0952) -> (-7.1726, -12.0756)
  line L109 (-7.1726, -12.0756) -> (-6.5261, -11.238)
  spline S42 degree 5 poles (-6.5261, -11.238) (-6.513, -11.2277) (-6.4867, -11.2076) (-6.4466, -11.1795) (-6.3921, -11.1459) (-6.3221, -11.1109) (-6.25, -11.0834) (-6.1756, -11.0641) (-6.099, -11.0534) (-6.0201, -11.0509) (-5.9392, -11.0559) (-5.8729, -11.0655) (-5.8224, -11.0756) (-5.7884, -11.0836) (-5.7713, -11.0879) knots 0 0 0 0 0 0 0.1 0.2 0.3 0.4 0.5 0.6 0.7 0.8 0.9 1 1 1 1 1 1
  arc A22 (-5.7713, -11.0879) -> (-5.2699, -11.3348) centre (0, 0) ccw
  spline S43 degree 5 poles (-5.2699, -11.3348) (-5.2579, -11.3455) (-5.2346, -11.3669) (-5.2014, -11.3998) (-5.1607, -11.4451) (-5.1162, -11.5042) (-5.0786, -11.5659) (-5.0486, -11.6305) (-5.0264, -11.6982) (-5.0117, -11.7688) (-5.0039, -11.842) (-5.0029, -11.9026) (-5.0047, -11.9491) (-5.0071, -11.9806) (-5.0086, -11.9964) knots -1 -1 -1 -1 -1 -1 -0.9 -0.8 -0.7 -0.6 -0.5 -0.4 -0.3 -0.2 -0.1 0 0 0 0 0 0
  line L110 (-5.0086, -11.9964) -> (-5.3939, -12.9192)
  line L111 (-5.3939, -12.9192) -> (-5.6489, -14.4382)
  line L112 (-5.6489, -14.4382) -> (-4.7261, -14.8235)
  line L113 (-4.7261, -14.8235) -> (-3.8028, -13.5206)
  line L114 (-3.8028, -13.5206) -> (-3.3951, -12.5442)
  spline S44 degree 5 poles (-3.3951, -12.5442) (-3.3852, -12.5308) (-3.3649, -12.5046) (-3.3335, -12.4671) (-3.2895, -12.4205) (-3.2309, -12.3685) (-3.1684, -12.3233) (-3.1016, -12.2855) (-3.0303, -12.2553) (-2.9548, -12.2325) (-2.8753, -12.2164) (-2.8088, -12.2085) (-2.7574, -12.2051) (-2.7225, -12.2041) (-2.7049, -12.2038) knots 0 0 0 0 0 0 0.1 0.2 0.3 0.4 0.5 0.6 0.7 0.8 0.9 1 1 1 1 1 1
  arc A23 (-2.7049, -12.2038) -> (-2.1566, -12.3126) centre (0, 0) ccw
  spline S45 degree 5 poles (-2.1566, -12.3126) (-2.1423, -12.3197) (-2.1143, -12.3344) (-2.0737, -12.3576) (-2.0226, -12.3908) (-1.9644, -12.4363) (-1.9121, -12.4862) (-1.8664, -12.5409) (-1.8274, -12.6005) (-1.7949, -12.6649) (-1.7685, -12.7337) (-1.7518, -12.7919) (-1.7415, -12.8373) (-1.7357, -12.8683) (-1.7331, -12.884) knots -1 -1 -1 -1 -1 -1 -0.9 -0.8 -0.7 -0.6 -0.5 -0.4 -0.3 -0.2 -0.1 0 0 0 0 0 0
  line L115 (-1.7331, -12.884) -> (-1.8664, -13.875)
  line L116 (-1.8664, -13.875) -> (-1.7195, -15.4083)
  line L117 (-1.7195, -15.4083) -> (-0.7284, -15.5416)
  line L118 (-0.7284, -15.5416) -> (-0.1738, -14.0441)
  line L119 (-0.1738, -14.0441) -> (0, -12.7519)
  line L120 (0, -12.7519) -> (0, -12.9212)
  spline S46 degree 5 poles (0, -12.9212) (0.0001, -12.921) (0.0073, -12.9063) (0.0221, -12.8775) (0.0458, -12.8358) (0.0804, -12.7833) (0.1291, -12.7235) (0.1838, -12.6697) (0.2448, -12.622) (0.3119, -12.5804) (0.3845, -12.5443) (0.4467, -12.5194) (0.4955, -12.5029) (0.5289, -12.4929) (0.5459, -12.4881) knots 0.098741 0.098741 0.098741 0.098741 0.098741 0.098741 0.1 0.2 0.3 0.4 0.5 0.6 0.7 0.8 0.9 1 1 1 1 1 1
  arc A24 (0.5459, -12.4881) -> (1.1036, -12.4512) centre (0, 0) ccw
  spline S47 degree 5 poles (1.1036, -12.4512) (1.1192, -12.4544) (1.1502, -12.4614) (1.1954, -12.4733) (1.2533, -12.4921) (1.3213, -12.521) (1.3847, -12.5557) (1.443, -12.5966) (1.4961, -12.6441) (1.5441, -12.6979) (1.5875, -12.7575) (1.6187, -12.8094) (1.6403, -12.8506) (1.654, -12.879) (1.6606, -12.8935) knots -1 -1 -1 -1 -1 -1 -0.9 -0.8 -0.7 -0.6 -0.5 -0.4 -0.3 -0.2 -0.1 0 0 0 0 0 0
  line L121 (1.6606, -12.8935) -> (1.7883, -13.8853)
  line L122 (1.7883, -13.8853) -> (2.3271, -15.3283)
  line L123 (0, 0) -> (0, -1.5)
  line L124 (0, -1.5) -> (0, 1.075)
  line L125 (0, 1.075) -> (1.0461, 1.075)
  line L126 (0, 1.075) -> (-1.0461, 1.075)
  dimension "d26" = 2.575
  constraint coincident A0.centre A1.centre
  constraint coincident A0 L123.end
  constraint vertical L123
  constraint parallel L123 L124
  constraint coincident A0 L125.end
  constraint perpendicular L124 L125
  constraint coincident A0 L126.end
  constraint perpendicular L124 L126
  measures "d26" distance of L123.end L124.end
extrude "Extrude3" add sketch "Sketch3" against normal blind 4 contours A0 L125 L126
extrude "Extrude4" add 1 faces at (-0.8856, 4, 8.6252) along direction (0, 1, 0) blind 1
